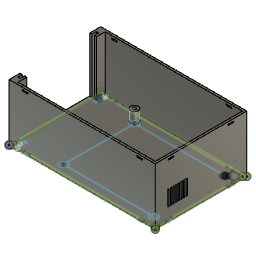
BOX (Autodesk Fusion 360 design; units mm, degrees)
Autodesk Fusion 360 part; units mm, degrees
sketch "Sketch1" plane through (0, 0, 0) normal (0, 0, 1) x (1, 0, 0)
  circle A0 centre (40.5, 74.5) radius 1.55
  circle A1 centre (40.5, 74.5) radius 3.5
  circle A2 centre (40.5, 9.5) radius 3.5
  circle A3 centre (40.5, 9.5) radius 1.55
  circle A4 centre (123.5, 74.5) radius 3.5
  circle A5 centre (123.5, 74.5) radius 1.55
  circle A6 centre (123.5, 9.5) radius 1.55
  circle A7 centre (123.5, 9.5) radius 3.5
  line L0 (123.5, 74.5) -> (40.5, 74.5)
  line L1 (123.5, 9.5) -> (40.5, 9.5)
  line L2 (40.5, 9.5) -> (40.5, 74.5)
  line L3 (0, 0) -> (134, 0)
  line L4 (134, 0) -> (134, 84)
  line L5 (134, 84) -> (0, 84)
  line L6 (0, 84) -> (0, 0)
  line L7 (2, 2) -> (132, 2)
  line L8 (132, 2) -> (132, 82)
  line L9 (132, 82) -> (2, 82)
  line L10 (2, 82) -> (2, 2)
  line L11 (132, 82) -> (123.5, 82)
  line L12 (123.5, 82) -> (123.5, 74.5)
  line L13 (123.5, 74.5) -> (132, 74.5)
  line L14 (132, 74.5) -> (132, 82)
  line L15 (2, 82) -> (4.2, 82)
  line L16 (4.2, 82) -> (4.2, 78)
  line L17 (4.2, 78) -> (2, 78)
  line L18 (2, 78) -> (2, 82)
  line L19 (4.2, 82) -> (6.2, 82)
  line L20 (6.2, 2) -> (4.2, 2)
  line L21 (2, 78) -> (4.2, 78)
  line L22 (4.2, 6) -> (2, 6)
  line L23 (2, 6) -> (2, 78)
  line L24 (4.2, 82) -> (6.2, 82)
  line L25 (6.2, 82) -> (6.2, 74)
  line L26 (6.2, 74) -> (4.2, 74)
  line L27 (4.2, 74) -> (4.2, 82)
  line L28 (4.2, 2) -> (6.2, 2)
  line L29 (6.2, 2) -> (6.2, 10)
  line L30 (6.2, 10) -> (4.2, 10)
  line L31 (4.2, 10) -> (4.2, 2)
  line L32 (2, 2) -> (0, 2)
  line L33 (0, 2) -> (0, 10)
  line L34 (0, 10) -> (2, 10)
  line L35 (2, 10) -> (2, 2)
  line L36 (2, 82) -> (0, 82)
  line L37 (0, 82) -> (0, 74)
  line L38 (0, 74) -> (2, 74)
  line L39 (2, 74) -> (2, 82)
  line L40 (2, 2) -> (12, 2)
  line L41 (12, 2) -> (17, 2)
  line L42 (17, 2) -> (17, 0)
  line L43 (17, 0) -> (12, 0)
  line L44 (12, 0) -> (12, 2)
  line L45 (12, 82) -> (17, 82)
  line L46 (17, 82) -> (17, 84)
  line L47 (17, 84) -> (12, 84)
  line L48 (12, 84) -> (12, 82)
  line L49 (132, 2) -> (122, 2)
  line L50 (132, 2) -> (132, 12)
  line L51 (132, 12) -> (134, 12)
  line L52 (134, 12) -> (134, 17)
  line L53 (134, 17) -> (132, 17)
  line L54 (132, 17) -> (132, 12)
  line L55 (122, 2) -> (117, 2)
  line L56 (117, 2) -> (117, 0)
  line L57 (117, 0) -> (122, 0)
  line L58 (122, 0) -> (122, 2)
  line L59 (132, 82) -> (132, 72)
  line L60 (132, 82) -> (122, 82)
  line L61 (122, 82) -> (117, 82)
  line L62 (117, 82) -> (117, 84)
  line L63 (117, 84) -> (122, 84)
  line L64 (122, 84) -> (122, 82)
  line L65 (132, 72) -> (134, 72)
  line L66 (134, 72) -> (134, 67)
  line L67 (134, 67) -> (132, 67)
  line L68 (132, 67) -> (132, 72)
  dimension "d11" = 3.1
  dimension "d12" = 7
  dimension "d20" = 7
  dimension "d21" = 3.1
  dimension "d22" = 7
  dimension "d23" = 3.1
  dimension "d24" = 3.1
  dimension "d25" = 7
  dimension "d80" = 83
  dimension "d82" = 65
  dimension "d83" = 134
  dimension "d84" = 84
  dimension "d87" = 130
  dimension "d88" = 80
  dimension "d89" = 8.5
  dimension "d90" = 7.5
  dimension "d91" = 2.2
  dimension "d92" = 4
  dimension "d93" = 2
  dimension "d94" = 2.2
  dimension "d95" = 72
  dimension "d96" = 2
  dimension "d97" = 8
  dimension "d98" = 2
  dimension "d99" = 8
  dimension "d111" = 10
  dimension "d112" = 5
  dimension "d113" = 10
  dimension "d114" = 10
  dimension "d115" = 5
  dimension "d116" = 2
  dimension "d117" = 10
  dimension "d118" = 10
  dimension "d119" = 5
  dimension "d120" = 2
  dimension "d121" = 5
  constraint concentric A0 A1
  constraint concentric A2 A3
  constraint concentric A4 A5
  constraint concentric A6 A7
  constraint coincident A4.centre A5.centre
  constraint coincident A0.centre A1.centre
  constraint coincident A6.centre A7.centre
  constraint horizontal L1
  constraint coincident A2.centre A3.centre
  constraint perpendicular L1 L2
  constraint horizontal L3
  constraint vertical L4
  constraint horizontal L5
  constraint vertical L6
  constraint coincident L3.start L6.end
  constraint horizontal L7
  constraint vertical L8
  constraint horizontal L9
  constraint vertical L10
  constraint horizontal L11
  constraint vertical L12
  constraint horizontal L13
  constraint vertical L14
  constraint vertical L16
  constraint horizontal L19
  constraint horizontal L20
  constraint horizontal L21
  constraint horizontal L22
  constraint vertical L23
  constraint horizontal L24
  constraint vertical L25
  constraint horizontal L26
  constraint vertical L27
  constraint horizontal L28
  constraint vertical L29
  constraint horizontal L30
  constraint vertical L31
  constraint horizontal L32
  constraint vertical L33
  constraint horizontal L34
  constraint vertical L35
  constraint coincident L6 L33.end
  constraint horizontal L36
  constraint vertical L37
  constraint horizontal L38
  constraint vertical L39
  constraint coincident L6 L37.end
  constraint perpendicular L10 L40
  constraint horizontal L41
  constraint vertical L42
  constraint horizontal L43
  constraint vertical L44
  constraint horizontal L45
  constraint vertical L46
  constraint horizontal L47
  constraint vertical L48
  constraint coincident L5 L46.end
  constraint coincident L9 L45.start
  constraint perpendicular L8 L49
  constraint perpendicular L7 L50
  constraint horizontal L51
  constraint vertical L52
  constraint horizontal L53
  constraint vertical L54
  constraint horizontal L55
  constraint vertical L56
  constraint horizontal L57
  constraint vertical L58
  constraint perpendicular L13 L59
  constraint perpendicular L59 L60
  constraint horizontal L61
  constraint vertical L62
  constraint horizontal L63
  constraint vertical L64
  constraint horizontal L65
  constraint vertical L66
  constraint horizontal L67
  constraint vertical L68
  measures "d11" diameter of A0
  measures "d12" diameter of A1
  measures "d20" diameter of A2
  measures "d21" diameter of A3
  measures "d22" diameter of A4
  measures "d23" diameter of A5
  measures "d24" diameter of A6
  measures "d25" diameter of A7
  measures "d80" distance of A4.centre A0.centre
  measures "d82" distance of A2.centre A0.centre
  measures "d83" distance of L3.start L3.end
  measures "d84" distance of L3.start L5.end
  measures "d87" distance of L7.start L7.end
  measures "d88" distance of L7.start L9.end
  measures "d89" distance of L8.end L11.end
  measures "d90" distance of L8.end L13.end
  measures "d91" distance of L9.end L15.end
  measures "d92" distance of L9.end L17.end
  measures "d93" distance of L15.end L19.end
  measures "d94" distance of L17.end L16.end
  measures "d95" distance of L17.end L22.end
  measures "d96" distance of L15.end L19.end
  measures "d97" distance of L15.end L26.end
  measures "d98" distance of L20.end L20.start
  measures "d99" distance of L20.end L30.end
  measures "d111" distance of L7.start L40.end
  measures "d112" distance of L40.end L41.end
  measures "d113" distance of L7.end L49.end
  measures "d114" distance of L7.end L50.end
  measures "d115" distance of L50.end L53.end
  measures "d116" distance of L49.end L57.end
  measures "d117" distance of L8.end L59.end
  measures "d118" distance of L8.end L60.end
  measures "d119" distance of L60.end L61.end
  measures "d120" distance of L59.end L65.end
  measures "d121" distance of L59.end L67.end
extrude "Extrude1" add sketch "Sketch1" along normal blind 2 contours A0 L0 L2 | A0 A1 L0 L2 | A0 A1 L0 L2 | A0 L0 L2 | A2 A3 L1 L2 | A2 A3 L1 L2 | A3 L1 L2 | A3 L1 L2 | A4 A5 L12 L13 | A4 L7 L8 L9 L10 L12 L13 L17 L21 L22 L23 L25 L26 L27 L29 L30 L31 L35 L39 L40 L41 L45 L49 L50 L54 L55 L59 L60 L61 L68 | A4 A5 L0 L13 | A4 L8 L9 L11 L12 L13 L14 L59 L60 | A4 A5 L0 L12 | A5 L12 L13 | A5 L0 L13 | L4 L5 L8 L9 L11 L14 L59 L60 L64 L65 | A5 L0 L12 | L4 L8 L65 L66 L67 L68 | L5 L9 L61 L62 L63 L64 | L4 L8 L53 L67 | L5 L9 L46 L62 | L4 L8 L51 L52 L53 L54 | L5 L9 L45 L46 L47 L48 | L3 L4 L7 L8 L49 L50 L51 L58 | L5 L6 L9 L15 L19 L24 L36 L48 | L9 L16 L19 L24 L25 L26 L27 | L3 L7 L55 L56 L57 L58 | L9 L10 L15 L16 L17 L18 L21 L27 L39 | L3 L7 L42 L56 | L6 L10 L18 L23 L36 L37 L38 L39 | L3 L7 L41 L42 L43 L44 | L6 L10 L23 L34 L38 | L3 L6 L7 L20 L28 L32 L40 L44 | L6 L10 L23 L32 L33 L34 L35 | L7 L20 L28 L29 L30 L31 L40 | L7 L10 L22 L31 L35 L40 | A6 | A7
extrude "Extrude2" add sketch "Sketch1" along normal blind 12 contours A0 A1 L0 L2 | A0 A1 L0 L2 | A2 A3 L1 L2 | A2 A3 L1 L2 | A4 A5 L12 L13 | A4 A5 L0 L13 | A4 A5 L0 L12 | A7
extrude "Extrude3" add sketch "Sketch1" along normal blind 52 contours L4 L5 L8 L9 L11 L14 L59 L60 L64 L65 | L4 L8 L65 L66 L67 L68 | L5 L9 L61 L62 L63 L64 | L4 L8 L53 L67 | L5 L9 L46 L62 | L4 L8 L51 L52 L53 L54 | L5 L9 L45 L46 L47 L48 | L3 L4 L7 L8 L49 L50 L51 L58 | L5 L6 L9 L15 L19 L24 L36 L48 | L9 L16 L19 L24 L25 L26 L27 | L3 L7 L55 L56 L57 L58 | L9 L10 L15 L16 L17 L18 L21 L27 L39 | L3 L7 L42 L56 | L6 L10 L18 L23 L36 L37 L38 L39 | L3 L7 L41 L42 L43 L44 | L3 L6 L7 L20 L28 L32 L40 L44 | L6 L10 L23 L32 L33 L34 L35 | L7 L20 L28 L29 L30 L31 L40 | L7 L10 L22 L31 L35 L40
sketch "Sketch6" plane through (134, 0, 0) normal (1, 0, 0) x (0, 1, 0)
  line L0 (0, 0) -> (84, 0)
  line L1 (84, 0) -> (84, 52)
  line L2 (84, 52) -> (0, 52)
  line L3 (0, 52) -> (0, 0)
  line L4 (0, 0) -> (11.5, 0)
  line L5 (11.5, 0) -> (11.5, 12)
  line L6 (11.5, 12) -> (0, 12)
  line L7 (0, 12) -> (0, 0)
  line L8 (11.5, 12) -> (29.5, 12)
  line L9 (29.5, 12) -> (29.5, 26)
  line L10 (29.5, 26) -> (11.5, 26)
  line L11 (11.5, 26) -> (11.5, 12)
  line L12 (11.5, 26) -> (12.7, 26)
  line L13 (12.7, 26) -> (12.7, 12)
  line L14 (12.7, 12) -> (11.5, 12)
  line L15 (11.5, 12) -> (11.5, 26)
  line L16 (13.9, 26) -> (13.9, 12)
  line L17 (15.1, 26) -> (15.1, 12)
  line L18 (16.3, 26) -> (16.3, 12)
  line L19 (17.5, 26) -> (17.5, 12)
  line L20 (18.7, 26) -> (18.7, 12)
  line L21 (19.9, 26) -> (19.9, 12)
  line L22 (21.1, 26) -> (21.1, 12)
  line L23 (22.3, 26) -> (22.3, 12)
  line L24 (23.5, 26) -> (23.5, 12)
  line L25 (24.7, 26) -> (24.7, 12)
  line L26 (25.9, 26) -> (25.9, 12)
  line L27 (27.1, 26) -> (27.1, 12)
  line L28 (28.3, 26) -> (28.3, 12)
  line L29 (29.5, 26) -> (29.5, 12)
  dimension "d100" = 11.5
  dimension "d101" = 12
  dimension "d102" = 18
  dimension "d103" = 14
  dimension "d104" = 1.2
  dimension "d107" = 16.8
  dimension "d108" = 0
  constraint horizontal L4
  constraint vertical L5
  constraint horizontal L6
  constraint vertical L7
  constraint coincident L0.start L3.end
  constraint horizontal L8
  constraint vertical L9
  constraint horizontal L10
  constraint vertical L11
  constraint horizontal L12
  constraint vertical L13
  constraint horizontal L14
  constraint vertical L15
  constraint coincident L8 L13.end
  measures "d100" distance of L0.start L4.end
  measures "d101" distance of L0.start L6.end
  measures "d102" distance of L5.end L8.end
  measures "d103" distance of L5.end L10.end
  measures "d104" distance of L10.end L12.end
extrude "Extrude6" cut sketch "Sketch6" against normal blind 2 contours L8 L10 L11 L12 L13 L14 L15 | L8 L10 L16 L17 | L8 L10 L18 L19 | L8 L10 L20 L21 | L8 L10 L22 L23 | L8 L10 L24 L25 | L8 L10 L26 L27 | L8 L9 L10 L28 L29
extrude "Extrude7" cut sketch "Sketch1" along normal blind 1 from surface at 49 contours L4 L8 L65 L66 L67 L68 | L5 L9 L61 L62 L63 L64 | L4 L8 L51 L52 L53 L54 | L5 L9 L45 L46 L47 L48 | L3 L7 L55 L56 L57 L58 | L3 L7 L41 L42 L43 L44
equation "d28 = 2 mm + 10.00 mm"
equation "d30 = 2 mm + 50 mm"
equation "d83 = 130 mm + ( 2 * 2 ) * 1 mm"
equation "d84 = 80 mm + ( 2 * 2 ) * 1 mm"
equation "d89 = 5 mm + ( 7 / 2 ) * 1 mm"
equation "d92 = 5 mm - 1 mm"
equation "d100 = 9.5 mm + 2 mm"
equation "d107 = 18.00 mm - 1.2 mm"
equation "d122 = 52 mm - 3 mm"
